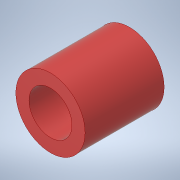
# Autodesk Inventor part: Spacer Creator
Saved by Autodesk Inventor 2022.3 (Build 263350000, 350)
## iProperties
Created: 2023-01-29
Part Number: Spacer Creator
Material: ABS Plastic
Document SubType Name: Modeling
Designer: mavericks
Density: 1.06 g/cm^3
Appearance: Smooth - Red
RuleStatus: InUse
AfterDocNew0: Open Form 1
Author: mavericks
Autodesk Inventor part; units mm, degrees
ref_plane "YZ Plane" through (0, 0, 0) normal (1, 0, 0) x (0, 1, 0)
ref_plane "XZ Plane" through (0, 0, 0) normal (0, 1, 0) x (-1, 0, 0)
ref_plane "XY Plane" through (0, 0, 0) normal (0, 0, 1) x (1, 0, 0)
sketch "Sketch1" plane through (0, 0, 0) normal (0, 0, 1) x (1, 0, 0)
  circle A0 centre (0, 0) radius 11.1125
  dimension "d10" = 22.225
  constraints: 2 coincident, 1 centre point
  measures "d10" diameter of A0
extrude "Extrusion1" add sketch "Sketch1" along normal blind 25.4
hole "Hole1" at (0, 0, 0) direction (0, 0, 1) diameter 13.8 end through all
equation "\"d10\" = OutsideDiameter"
equation "\"d1\" = SpacerLength"
equation "\"d3\" = HoleDiameter"
equation "\"SpacerLength\" = 25.4"
equation "\"HoleDiameter\" = 13.8"
equation "\"OutsideDiameter\" = 22.225"
body "Solid1"
